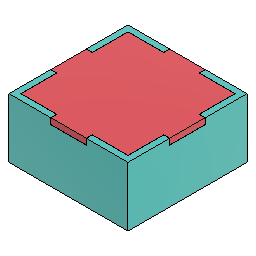
Scatola_parametrica_configurabile (Autodesk Fusion 360 archive; units mm, degrees)
design "Scatola_parametrica_configurabile"
part number: 100
Autodesk Fusion 360 part; units mm, degrees
sketch "Schizzo1" plane through (0, 0, 0) normal (0, 0, 1) x (1, 0, 0) in component "Base"
  line L0 (50, 50) -> (-50, 50)
  line L1 (-50, 50) -> (-50, -50)
  line L2 (-50, -50) -> (50, -50)
  line L3 (50, -50) -> (50, 50)
  line L4 (50, 50) -> (-50, -50) construction
  line L5 (-50, 50) -> (50, -50) construction
  dimension "d9" = 100
  dimension "d10" = 100
  constraint horizontal L0
  constraint perpendicular L0 L1
  constraint parallel L0 L2
  constraint parallel L1 L3
  constraint coincident L4 origin
  constraint coincident L5 origin
  measures "d9" distance of L0.start L0.end
  measures "d10" distance of L0.end L1.end
extrude "Estrusione1" add sketch "Schizzo1" along normal blind 50 makes body 1 in component "Base"
shell "Svuotamento2" thickness 5 removed faces 1 at (16.6667, -16.6667, 50) on bodies 1 in component "Base"
sketch "Schizzo2" plane through (0, 0, 50) normal (0, 0, 1) x (-1, 0, 0) in component "Base"
  line L0 (-45, 45) -> (45, 45)
  line L1 (45, 45) -> (45, -45)
  line L2 (45, -45) -> (-45, -45)
  line L3 (-45, -45) -> (-45, 45)
  line L4 (-50, 50) -> (-50, -50)
  line L5 (-50, -50) -> (50, -50)
  line L6 (50, -50) -> (50, 50)
  line L7 (50, 50) -> (-50, 50)
  line L8 (15, -50) -> (-15, -50)
  line L9 (-15, -50) -> (-15, -45)
  line L10 (-15, -45) -> (15, -45)
  line L11 (15, -45) -> (15, -50)
  line L12 (-50, -15) -> (-45, -15)
  line L13 (-45, -15) -> (-45, 15)
  line L14 (-45, 15) -> (-50, 15)
  line L15 (-50, 15) -> (-50, -15)
  line L16 (15, 45) -> (-15, 45)
  line L17 (-15, 45) -> (-15, 50)
  line L18 (-15, 50) -> (15, 50)
  line L19 (15, 50) -> (15, 45)
  line L20 (50, -15) -> (45, -15)
  line L21 (45, -15) -> (45, 15)
  line L22 (45, 15) -> (50, 15)
  line L23 (50, 15) -> (50, -15)
  line L24 (0, -1.75) -> (0, -22.5)
  line L25 (-1.75, 0) -> (-22.5, 0)
  dimension "d15" = 30
  constraint horizontal L8
  constraint vertical L9
  constraint horizontal L10
  constraint vertical L11
  constraint coincident L2 L9.end
  constraint coincident L5 L8.start
  constraint horizontal L12
  constraint vertical L13
  constraint horizontal L14
  constraint vertical L15
  constraint coincident L3 L13.end
  constraint coincident L4 L12.start
  constraint horizontal L16
  constraint vertical L17
  constraint horizontal L18
  constraint vertical L19
  constraint coincident L7 L17.end
  constraint coincident L0 L16.start
  constraint horizontal L20
  constraint vertical L21
  constraint horizontal L22
  constraint vertical L23
  constraint coincident L1 L21.end
  constraint coincident L6 L20.start
  constraint symmetric L9 L11 L24
  constraint symmetric L20 L22 L25
  constraint symmetric L12 L14 L25
  constraint symmetric L17 L19 L24
  constraint equal L8 L23
  constraint equal L8 L15
  constraint equal L8 L18
  measures "d15" distance of L8.start L8.end
extrude "Estrusione2" cut sketch "Schizzo2" against normal blind 5 contours L0 L7 L16 L17 L18 L19 | L3 L4 L12 L13 L14 L15 | L1 L6 L20 L21 L22 L23 | L2 L5 L8 L9 L10 L11 bodies 1 in component "Base"
sketch "Schizzo2 (2)" plane through (0, 0, 45) normal (0, 0, 1) x (-1, 0, 0) in component "Coperchio"
  line L0 (15, 50) -> (-15, 50) construction
  line L1 (-15, 50) -> (-15, 45) construction
  line L2 (15, 45) -> (15, 50) construction
  line L3 (15, -50) -> (-15, -50) construction
  line L4 (15, -45) -> (15, -50) construction
  line L5 (45, -45) -> (15, -45) construction
  line L6 (45, -15) -> (45, -45) construction
  line L7 (50, -15) -> (45, -15) construction
  line L8 (50, 15) -> (50, -15) construction
  line L9 (45, 15) -> (50, 15) construction
  line L10 (45, 45) -> (45, 15) construction
  line L11 (15, 45) -> (45, 45) construction
  line L12 (15, 50) -> (15, 45) construction
  line L13 (-15, 50) -> (15, 50) construction
  line L14 (-15, 45) -> (-15, 50) construction
  line L15 (-45, 45) -> (-15, 45) construction
  line L16 (-45, 15) -> (-45, 45) construction
  line L17 (-50, 15) -> (-45, 15) construction
  line L18 (-50, -15) -> (-50, 15) construction
  line L19 (-45, -15) -> (-50, -15) construction
  line L20 (-45, -45) -> (-45, -15) construction
  line L21 (-15, -45) -> (-45, -45) construction
  line L22 (-15, -50) -> (-15, -45) construction
  line L23 (50, -15) -> (45, -15) construction
  line L24 (45, -15) -> (45, -45) construction
  line L25 (45, -45) -> (15, -45) construction
  line L26 (15, -45) -> (15, -50) construction
  line L27 (-49.9, -14.9) -> (-49.9, 14.9)
  line L28 (-49.9, 14.9) -> (-44.9, 14.9)
  line L29 (-44.9, 14.9) -> (-44.9, 44.9)
  line L30 (-44.9, 44.9) -> (-14.9, 44.9)
  line L31 (-14.9, 44.9) -> (-14.9, 49.9)
  line L32 (-14.9, 49.9) -> (14.9, 49.9)
  line L33 (14.9, 49.9) -> (14.9, 44.9)
  line L34 (14.9, 44.9) -> (44.9, 44.9)
  line L35 (44.9, 44.9) -> (44.9, 14.9)
  line L36 (44.9, 14.9) -> (49.9, 14.9)
  line L37 (49.9, 14.9) -> (49.9, -14.9)
  line L38 (49.9, -14.9) -> (44.9, -14.9)
  line L39 (44.9, -14.9) -> (44.9, -44.9)
  line L40 (44.9, -44.9) -> (14.9, -44.9)
  line L41 (14.9, -44.9) -> (14.9, -49.9)
  line L42 (14.9, -49.9) -> (-14.9, -49.9)
  line L43 (-14.9, -49.9) -> (-14.9, -44.9)
  line L44 (-14.9, -44.9) -> (-44.9, -44.9)
  line L45 (-44.9, -44.9) -> (-44.9, -14.9)
  line L46 (-44.9, -14.9) -> (-49.9, -14.9)
  dimension "d18" = 0.1
extrude "Estrusione1'" add sketch "Schizzo2 (2)" along normal up to surface (5 mm away) separate body makes body 2 in component "Coperchio"
component "Base" placed x (1, 0, 0) y (0, 1, 0) z (0, 0, 1) at (0, 0, 0)
component "Coperchio" placed x (1, 0, 0) y (0, -1, 0) z (0, 0, -1) at (0, 0, 95)
equation "Larghezza_Base = 100 mm"
equation "Profondità = 100 mm"
equation "Altezza = 50 mm"
equation "Spessore = 5 mm"
equation "d9 = Larghezza_Base"
equation "d10 = Profondità"
equation "d11 = Altezza"
equation "d14 = Spessore"
equation "d16 = -Spessore"
